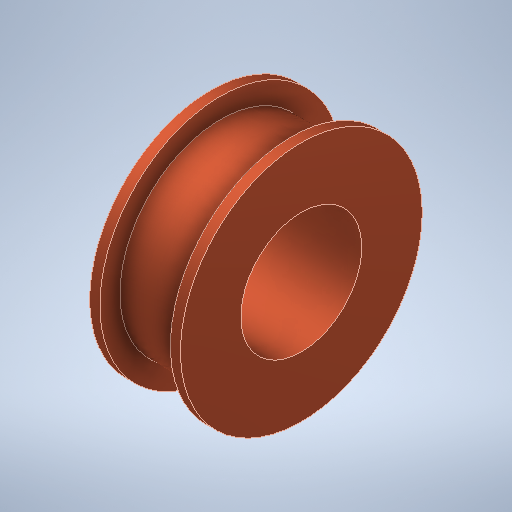
# Autodesk Inventor part: 202 part 2
Saved by Autodesk Inventor 2025.1 (Build 291241000, 241)
## iProperties
Created: 2024-09-02
Part Number: 202 part 2
Material: Copper, Alloy
Document SubType Name: Modeling
Designer: ffogue
Density: 8.92 g/cm^3
Appearance: Copper - Satin
Author: ffogue
Autodesk Inventor part; units mm, degrees
ref_plane "YZ Plane" through (0, 0, 0) normal (1, 0, 0) x (0, 1, 0)
ref_plane "XZ Plane" through (0, 0, 0) normal (0, 1, 0) x (-1, 0, 0)
ref_plane "XY Plane" through (0, 0, 0) normal (0, 0, 1) x (1, 0, 0)
sketch "Sketch1" plane through (0, 0, 0) normal (0, 0, 1) x (1, 0, 0)
  line L0 (0, 0) -> (0, 12)
  line L1 (0, 12) -> (1, 12)
  line L2 (1, 12) -> (1, 10)
  line L3 (1, 10) -> (8, 10)
  line L4 (8, 10) -> (8, 12)
  line L5 (8, 12) -> (9, 12)
  line L6 (9, 12) -> (9, 0)
  line L7 (9, 0) -> (0, 0)
  dimension "d1" = 9
  dimension "d2" = 7
  dimension "d3" = 20
  dimension "d4" = 24
  dimension "d13" = 1
  constraints: 16 end point, 5 perpendicular, 2 point on line, 1 parallel, 1 vertical
  measures "d1" distance between parallel lines of L6 L0
  measures "d2" distance of L2.end L3.end
  measures "d3" diameter of L3 L7
  measures "d4" diameter of L5 L7
  measures "d13" distance of L0.end L1.end
revolve "Revolution1" add sketch "Sketch1" angle 360 about axis through (9, 0, 0) along (-1, 0, 0)
sketch "Sketch2" plane through (9, 0, 0) normal (1, 0, 0) x (0, 0, -1)
  circle A0 centre (0, 0) radius 12 projected
  constraints: 1 coincident
hole "Hole1" at (9, 0, 0) direction (-1, 0, 0) diameter 12 depth 9
body "Solid1"
